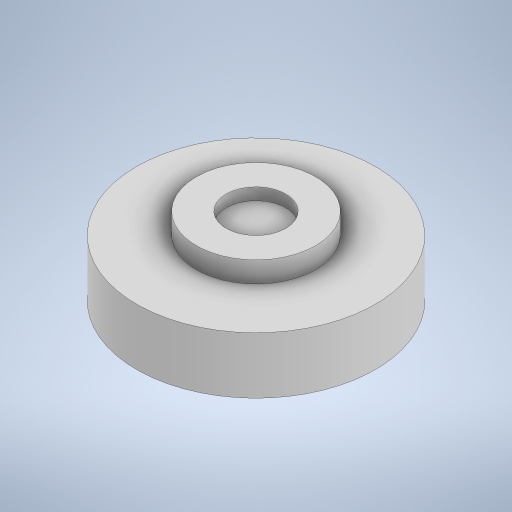
# Autodesk Inventor part: part6
Saved by Autodesk Inventor 2024 (Build 280153000, 153)
## iProperties
Created: 2023-08-22
Part Number: part6
Material: Generic
Document SubType Name: Modeling
Designer: admins
Density: 1 g/cm^3
Appearance: Default
Author: admins
Autodesk Inventor part; units mm, degrees
ref_plane "YZ Plane" through (0, 0, 0) normal (1, 0, 0) x (0, 1, 0)
ref_plane "XZ Plane" through (0, 0, 0) normal (0, 1, 0) x (-1, 0, 0)
ref_plane "XY Plane" through (0, 0, 0) normal (0, 0, 1) x (1, 0, 0)
sketch "Sketch1" plane through (0, 0, 0) normal (0, 1, 0) x (-1, 0, 0)
  circle A0 centre (12.7112, 19.8484) radius 40
  point P0 (0, 0)
  constraints: 1 centre point
extrude "Extrusion1" add sketch "Sketch1" along normal blind 19
sketch "Sketch2" plane through (-12.7112, 19, 19.8484) normal (0, 1, 0) x (1, 0, 0)
  point P0 (12.7112, 19.8484)
sketch "Sketch3" plane through (-12.7112, 19, 19.8484) normal (0, 1, 0) x (1, 0, 0)
  circle A0 centre (0, 0) radius 20
  point P0 (12.7112, 19.8484)
  dimension "d3" = 40
  constraints: 1 centre point
  measures "d3" diameter of A0
extrude "Extrusion2" add sketch "Sketch3" along normal blind 7
sketch "Sketch4" plane through (-12.7112, 26, 19.8484) normal (0, 1, 0) x (1, 0, 0)
  circle A0 centre (0, 0) radius 10
  point P0 (12.7112, 19.8484)
  dimension "d6" = 20
  constraints: 1 centre point
  measures "d6" diameter of A0
extrude "Extrusion3" cut sketch "Sketch4" against normal blind 4
body "Solid1"
